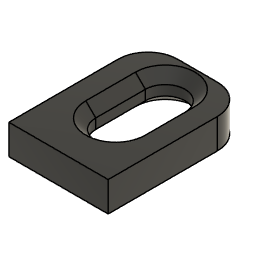
86e05428-901b-4174-a4a0-95a3f9a26929 (Autodesk Fusion 360 design; units mm, degrees)
Autodesk Fusion 360 part; units mm, degrees
sketch "Esboço1" plane through (0, -30.8571, 0) normal (0, -1, 0) x (1, 0, 0)
  line L0 (-10.6636, -6.4303) -> (-0.6636, -6.4303)
  line L1 (-0.6636, -6.4303) -> (-0.6636, -3.4303)
  line L2 (-0.6636, -3.4303) -> (-10.6636, -3.4303)
  line L3 (-10.6636, -3.4303) -> (-10.6636, -6.4303)
  line L4 (-10.6636, -6.4303) -> (-0.6636, -6.4303)
  line L5 (-0.6636, -6.4303) -> (-0.6636, 4.5697)
  line L6 (-3.6636, 7.5697) -> (-7.6636, 7.5697)
  line L7 (-10.6636, 4.5697) -> (-10.6636, -6.4303)
  line L8 (-5.6636, -6.4303) -> (-5.6636, 7.5697) construction
  line L9 (-3.6636, 4.3197) -> (-3.6636, -0.6803)
  line L10 (-7.6636, 4.3197) -> (-7.6636, -0.6803)
  arc A0 (-3.6636, 4.3197) -> (-7.6636, 4.3197) centre (-5.6636, 4.3197) ccw
  arc A1 (-7.6636, -0.6803) -> (-3.6636, -0.6803) centre (-5.6636, -0.6803) ccw
  arc A2 (-7.6636, 7.5697) -> (-10.6636, 4.5697) centre (-7.6636, 4.5697) ccw
  arc A3 (-0.6636, 4.5697) -> (-3.6636, 7.5697) centre (-3.6636, 4.5697) ccw
  point P0 (-0.6636, 7.5697)
  dimension "d641" = 14
  dimension "d642" = 10
  dimension "d643" = 5
  dimension "d645" = 4
  dimension "d646" = 3
  dimension "d647" = 3.25
  constraint horizontal L4
  constraint vertical L5
  constraint horizontal L6
  constraint vertical L7
  constraint coincident L0.start L3.end
  constraint midpoint L4 L8.start
  constraint coincident L8 A0.centre
  constraint coincident L8 A1.centre
  constraint equal A0 A1
  constraint parallel L8 L9
  constraint vertical L10
  constraint tangent L10 A0
  constraint tangent L9 A0
  constraint coincident L6 L8.end
  constraint tangent L6 A2
  constraint tangent L7 A2
  constraint coincident P0 L6
  constraint coincident P0 L5
  constraint tangent L6 A3
  constraint tangent L5 A3
  constraint equal A2 A3
  measures "d641" distance of L0.end P0
  measures "d642" distance of L0.start L0.end
  measures "d643" distance of A0.centre A1.centre
  measures "d645" diameter of A0
  measures "d646" radius of A2
  measures "d647" distance of L6 A0.centre
extrude "Extrusão1" add sketch "Esboço1" along normal blind 3
chamfer "Chanfro1" distance 1 angle 45 8 edges at (-7.6636, -33.8571, 1.8197) (-5.6636, -33.8571, 6.3197) (-3.6636, -33.8571, 1.8197) (-5.6636, -33.8571, -2.6803) (-7.6636, -30.8571, 1.8197) (-5.6636, -30.8571, 6.3197) (-3.6636, -30.8571, 1.8197) (-5.6636, -30.8571, -2.6803)
move_body "Mover1" bodies 1 to x (1, 0, 0) y (0, 0, -1) z (0, 1, 0) at (0, -37.1769, -28.5374)
